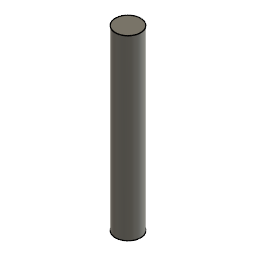
OTIS model assembly (Autodesk Fusion 360 archive; units mm, degrees)
design "Front wheel shaft"
part number: 2026-08-01-14-16-07-346
Autodesk Fusion 360 part; units mm, degrees
sketch "Sketch1" plane through (0, 0, 0) normal (0, 1, 0) x (1, 0, 0)
  circle A0 centre (0, 0) radius 1
  dimension "d1" = 2
  constraint coincident A0.centre origin
  measures "d1" diameter of A0
extrude "Extrude1" add sketch "Sketch1" along normal blind 14

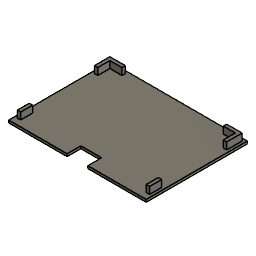
design "OTIS roof"
part number: 2026-08-06-09-41-14-601
Autodesk Fusion 360 part; units mm, degrees
sketch "Sketch1" plane through (0, 0, 0) normal (0, 1, 0) x (1, 0, 0)
  line L0 (0, 0) -> (80, 0)
  line L1 (80, 0) -> (80, 58.89)
  line L2 (80, 58.89) -> (0, 58.89)
  line L3 (0, 58.89) -> (0, 0)
  line L4 (46, 0) -> (34, 0)
  line L5 (34, 0) -> (34, 8)
  line L6 (34, 8) -> (46, 8)
  line L7 (46, 8) -> (46, 0)
  dimension "d1" = 58.89
  dimension "d2" = 80
  dimension "d11" = 8
  dimension "d14" = 12
  dimension "d15" = 34
  constraint horizontal L0
  constraint vertical L1
  constraint horizontal L2
  constraint vertical L3
  constraint coincident L0.start L3.end
  constraint horizontal L4
  constraint vertical L5
  constraint horizontal L6
  constraint vertical L7
  constraint coincident L0 L4.start
  measures "d1" distance of L0.start L2.end
  measures "d2" distance of L1 L3
  measures "d11" distance of L4.end L5.end
  measures "d14" distance of L5.end L6.end
  measures "d15" distance of L3 L5
extrude "Extrude1" add sketch "Sketch1" along normal blind 1.5
sketch "Sketch2" plane through (0, 1.5, 0) normal (0, 1, 0) x (-1, 0, 0)
  line L0 (0, -58.89) -> (0, 0)
  line L1 (0, 0) -> (-80, 0)
  line L2 (-80, 0) -> (-80, -58.89)
  line L3 (-80, -58.89) -> (0, -58.89)
  line L4 (-10.51, -1.51) -> (-1.51, -1.51)
  line L5 (-1.51, -1.51) -> (-1.51, -10.51)
  line L6 (-1.51, -10.51) -> (-10.51, -10.51)
  line L7 (-10.51, -10.51) -> (-10.51, -1.51)
  line L8 (-10.51, -10.51) -> (-3.51, -10.51)
  line L9 (-3.51, -10.51) -> (-3.51, -3.51)
  line L10 (-3.51, -3.51) -> (-10.51, -3.51)
  line L11 (-10.51, -3.51) -> (-10.51, -10.51)
  line L12 (0, -29.445) -> (-80, -29.445) construction
  line L13 (-3.51, -48.38) -> (-3.51, -55.38)
  line L14 (-3.51, -55.38) -> (-10.51, -55.38)
  line L15 (-10.51, -48.38) -> (-10.51, -57.38)
  line L16 (-1.51, -48.38) -> (-10.51, -48.38)
  line L17 (-1.51, -57.38) -> (-1.51, -48.38)
  line L18 (-10.51, -57.38) -> (-1.51, -57.38)
  line L19 (-69.49, -1.51) -> (-78.49, -1.51)
  line L20 (-76.49, -3.51) -> (-69.49, -3.51)
  line L21 (-78.49, -1.51) -> (-78.49, -10.51)
  line L22 (-76.49, -10.51) -> (-76.49, -3.51)
  line L23 (-78.49, -10.51) -> (-69.49, -10.51)
  line L24 (-69.49, -10.51) -> (-69.49, -1.51)
  line L25 (-78.49, -48.38) -> (-69.49, -48.38)
  line L26 (-69.49, -48.38) -> (-69.49, -57.38)
  line L27 (-76.49, -48.38) -> (-76.49, -55.38)
  line L28 (-78.49, -57.38) -> (-78.49, -48.38)
  line L29 (-76.49, -55.38) -> (-69.49, -55.38)
  line L30 (-69.49, -57.38) -> (-78.49, -57.38)
  line L31 (-3.51, -3.51) -> (-1.51, -3.51)
  line L32 (-76.49, -3.51) -> (-78.49, -3.51)
  dimension "d5" = 9
  dimension "d6" = 9
  dimension "d7" = 1.51
  dimension "d8" = 1.51
  constraint horizontal L4
  constraint vertical L5
  constraint horizontal L6
  constraint vertical L7
  constraint horizontal L8
  constraint vertical L9
  constraint horizontal L10
  constraint vertical L11
  constraint coincident L5 L31.end
  constraint perpendicular L9 L31
  constraint coincident L21 L32.end
  constraint perpendicular L21 L32
  measures "d5" distance of L4.start L4.end
  measures "d6" distance of L4.start L6.end
  measures "d7" distance of L0 L5
  measures "d8" distance of L1 L4
extrude "Extrude2" add sketch "Sketch2" along normal blind 4 contours L5 L6 L9 L31 | L13 L14 L15 L16 L17 L18 | L21 L22 L23 L32 | L25 L26 L27 L28 L29 L30
extrude "Extrude3" cut sketch "Sketch1" along normal blind 8.263 contours L0 L4 L5 L6 L7

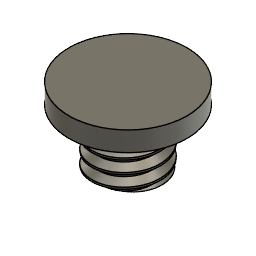
design "M2.5 x 6mm Phillips Flat Head Screw"
part number: 2026-08-01-20-11-09-453
Autodesk Fusion 360 part; units mm, degrees
sketch "Sketch1" plane through (0, 0, 0) normal (0, 1, 0) x (1, 0, 0)
  circle A0 centre (0, 0) radius 1.5
  dimension "d1" = 3
  constraint coincident A0.centre origin
  measures "d1" diameter of A0
extrude "Extrude1" add sketch "Sketch1" along normal blind 2
thread "Thread1" "ISO Metric profile 2.5 M2.5x0.45 M2.5x0.45 6g" major diameter 2.43 minor diameter 1.9165 pitch 0.45 angle 60 modelled right hand crest width 0.0648 on face at (1.4981, 1.3333, 0.0748) crest through (1.215, -0.1125, 0)
sketch "Sketch2" plane through (0, 2, 0) normal (0, 1, 0) x (-1, 0, 0)
  spline S0 degree 3 poles (-0.1252, 1.2085) (-0.2764, 1.1771) (-0.4201, 1.117) (-0.6707, 0.9476) (-0.7764, 0.8419) (-0.9369, 0.6004) (-0.9921, 0.4683) (-1.0464, 0.1962) (-1.0473, 0.0593) (-1.0042, -0.1619) (-0.9753, -0.2474) (-0.8966, -0.4057) (-0.8477, -0.4781) (-0.7897, -0.5428) knots 0 0 0 0 0.046326 0.046326 0.090815 0.090815 0.133466 0.133466 0.17428 0.17428 0.201332 0.201332 0.227524 0.227524 0.227524 0.227524
  arc A0 (-0.7897, -0.5428) -> (0.2561, -0.9234) centre (0, 0) ccw
  spline S1 degree 3 poles (0.2561, -0.9234) (0.3815, -0.9055) (0.5022, -0.8627) (0.7262, -0.7312) (0.8263, -0.6416) (0.9913, -0.4249) (1.0527, -0.2985) (1.1264, -0.0233) (1.1356, 0.1233) (1.1038, 0.3714) (1.0763, 0.4727) (0.9942, 0.6681) (0.9393, 0.7609) (0.8727, 0.8453) knots 0 0 0 0 0.038021 0.038021 0.077873 0.077873 0.119555 0.119555 0.163068 0.163068 0.19429 0.19429 0.22638 0.22638 0.22638 0.22638
  arc A1 (0.8727, 0.8453) -> (-0.1252, 1.2085) centre (0, 0) ccw
  circle A2 centre (0, 0) radius 2.1
  dimension "d6" = 4.2
  constraint coincident A0.centre A1.centre
  measures "d6" diameter of A2
extrude "Extrude2" add sketch "Sketch2" along normal blind 0.7 contours S0 A0 S1 A1 | A2

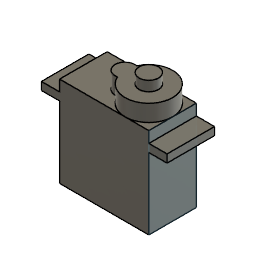
design "MG90S servo model"
part number: 2026-07-24-13-32-31-393
Autodesk Fusion 360 part; units mm, degrees
sketch "Sketch1" plane through (0, 0, 0) normal (0, 1, 0) x (1, 0, 0)
  line L0 (0, 0) -> (22.5, 0)
  line L1 (22.5, 0) -> (22.5, 12)
  line L2 (22.5, 12) -> (0, 12)
  line L3 (0, 12) -> (0, 0)
  dimension "d1" = 22.5
  dimension "d2" = 12
  constraint horizontal L0
  constraint vertical L1
  constraint horizontal L2
  constraint vertical L3
  constraint coincident L0.start L3.end
  measures "d1" distance of L0.start L0.end
  measures "d2" distance of L0.start L2.end
extrude "Extrude1" add sketch "Sketch1" along normal blind 22.8
sketch "Sketch2" plane through (22.5, 0, 0) normal (1, 0, 0) x (0, 0, -1)
  line L0 (0, 0) -> (12, 0)
  line L1 (12, 0) -> (12, 22.8)
  line L2 (12, 22.8) -> (0, 22.8)
  line L3 (0, 22.8) -> (0, 0)
sketch "Sketch3" plane through (0, 22.8, 0) normal (0, 1, 0) x (-1, 0, 0)
  line L0 (0, -12) -> (0, 0)
  line L1 (0, 0) -> (-22.5, 0)
  line L2 (-22.5, 0) -> (-22.5, -12)
  line L3 (-22.5, -12) -> (0, -12)
  line L4 (-22.5, -6) -> (-16.5, -6) construction
  circle A0 centre (-16.5, -6) radius 6
  line L5 (-16.5, -6) -> (0, -6) construction
  circle A1 centre (-10.5, -6) radius 2.5
  dimension "d5" = 6
  dimension "d6" = 12
  dimension "d16" = 5
  constraint midpoint L2 L4.start
  constraint perpendicular L2 L4
  constraint coincident L4.end A0.centre
  constraint midpoint L0 L5.end
  constraint coincident A0 A1.centre
  constraint coincident L5 A1.centre
  measures "d5" distance of L4.start L4.end
  measures "d6" diameter of A0
  measures "d16" diameter of A1
extrude "Extrude2" add sketch "Sketch3" along normal blind 4.2 contours A0 A1 | A0 A1 | A0 A1
sketch "Sketch4" plane through (0, 27, 0) normal (0, 1, 0) x (-1, 0, 0)
  arc A0 (-11.0208, -8.4451) -> (-11.0208, -3.5549) centre (-10.5, -6) ccw
  arc A1 (-11.0208, -3.5549) -> (-11.0208, -8.4451) centre (-16.5, -6) ccw
  circle A2 centre (-16.5, -6) radius 2.45
  dimension "d17" = 4.9
  constraint concentric A1 A2
  measures "d17" diameter of A2
sketch "Sketch5" plane through (22.5, 0, 0) normal (1, 0, 0) x (0, 0, -1)
  line L0 (12, 18) -> (0, 18)
  line L1 (0, 18) -> (0, 20)
  line L2 (0, 20) -> (12, 20)
  line L3 (12, 20) -> (12, 18)
  constraint horizontal L0
  constraint vertical L1
  constraint horizontal L2
  constraint vertical L3
extrude "Extrude4" add sketch "Sketch5" along normal blind 4.6
sketch "Sketch8" plane through (0, 0, 0) normal (-1, 0, 0) x (0, 0, 1)
  line L0 (-12, 0) -> (0, 0)
  line L1 (0, 0) -> (0, 22.8)
  line L2 (0, 22.8) -> (-12, 22.8)
  line L3 (-12, 22.8) -> (-12, 0)
  line L4 (-12, 20) -> (0, 20)
  line L5 (0, 20) -> (0, 18)
  line L6 (0, 18) -> (-12, 18)
  line L7 (-12, 18) -> (-12, 20)
extrude "Extrude5" add sketch "Sketch8" along normal blind 4.6 contours L1 L3 L4 L5 L6 L7
extrude "Extrude6" add sketch "Sketch4" along normal blind 2.5 contours A2

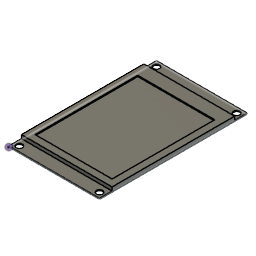
design "rough 2.4 in lcd model"
part number: 2026-07-24-14-02-43-553
Autodesk Fusion 360 part; units mm, degrees
sketch "Sketch1" plane through (0, 0, 0) normal (0, 1, 0) x (1, 0, 0)
  line L0 (0, 0) -> (43.3, 0)
  line L1 (43.3, 0) -> (43.3, 70.5)
  line L2 (43.3, 70.5) -> (0, 70.5)
  line L3 (0, 70.5) -> (0, 0)
  dimension "d1" = 43.3
  dimension "d2" = 70.5
  constraint horizontal L0
  constraint vertical L1
  constraint horizontal L2
  constraint vertical L3
  constraint coincident L0.start L3.end
  measures "d1" distance of L0.start L0.end
  measures "d2" distance of L0.start L2.end
extrude "Extrude1" add sketch "Sketch1" along normal blind 0.5
sketch "Sketch2" plane through (0, 0.5, 0) normal (0, 1, 0) x (-1, 0, 0)
  line L0 (0, -70.5) -> (0, 0)
  line L1 (0, 0) -> (-43.3, 0)
  line L2 (-43.3, 0) -> (-43.3, -70.5)
  line L3 (-43.3, -70.5) -> (0, -70.5) construction
  line L4 (-43.3, 0) -> (-43.3, -5) construction
  line L5 (-43.3, -70.5) -> (-43.3, -64.5) construction
  line L6 (-43.3, -64.5) -> (0, -64.5)
  line L7 (0, -64.5) -> (0, -6)
  line L8 (0, -6) -> (-43.3, -6)
  line L9 (-43.3, -6) -> (-43.3, -64.5)
  line L10 (0, -2.5) -> (-2.5, -2.5) construction
  line L11 (-43.3, -2.5) -> (-40.8, -2.5) construction
  circle A0 centre (-2.5, -68) radius 1.5
  circle A1 centre (-40.8, -68) radius 1.5
  circle A2 centre (-40.8, -2.5) radius 1.5
  circle A3 centre (-2.5, -2.5) radius 1.5
  dimension "d5" = 6
  dimension "d8" = 2.5
  dimension "d10" = 3
  dimension "d11" = 3
  dimension "d12" = 3
  dimension "d13" = 3
  dimension "d16" = 2.5
  dimension "d17" = 2.5
  dimension "d18" = 2.5
  dimension "d19" = 2.5
  dimension "d20" = 2.5
  dimension "d21" = 2.5
  dimension "d22" = 2.5
  constraint coincident L1.end L2.start
  constraint coincident L2 L4.end
  constraint coincident L2.end L3.start
  constraint perpendicular L3 L5
  constraint horizontal L6
  constraint vertical L7
  constraint horizontal L8
  constraint vertical L9
  constraint coincident L0 L7.end
  constraint coincident L0 L10.start
  constraint perpendicular L0 L10
  constraint midpoint L4 L11.start
  constraint perpendicular L4 L11
  constraint coincident L11.end A2.centre
  constraint coincident L10.end A3.centre
  measures "d5" distance of L2.end L5.end
  measures "d8" distance of L11.start L11.end
  measures "d10" diameter of A0
  measures "d11" diameter of A1
  measures "d12" diameter of A2
  measures "d13" diameter of A3
  measures "d16" distance of L10.start L10.end
  measures "d17" distance of L1 L10.end
  measures "d18" distance of L1 L11.end
  measures "d19" distance of L5 A1.centre
  measures "d20" distance of L3 A1.centre
  measures "d21" distance of L3 A0.centre
  measures "d22" distance of L0 A0.centre
extrude "Extrude2" add sketch "Sketch2" along normal blind 1.67 contours L0 L2 L6 L7 L8 L9
extrude "Extrude3" cut sketch "Sketch2" against normal blind 5.737 contours A0 | A1 | A2 | A3
sketch "Sketch3" plane through (0, 2.17, 0) normal (0, 1, 0) x (-1, 0, 0)
  line L0 (-43.3, -6) -> (-43.3, -64.5)
  line L1 (-43.3, -64.5) -> (0, -64.5)
  line L2 (0, -64.5) -> (0, -6)
  line L3 (0, -6) -> (-43.3, -6)
  line L4 (-3.29, -9.29) -> (-40.01, -9.29)
  line L5 (-40.01, -9.29) -> (-40.01, -58.25)
  line L6 (-40.01, -58.25) -> (-3.29, -58.25)
  line L7 (-3.29, -58.25) -> (-3.29, -9.29)
  dimension "d23" = 36.72
  dimension "d24" = 48.96
  dimension "d25" = 3.29
  dimension "d26" = 3.29
  constraint horizontal L4
  constraint vertical L5
  constraint horizontal L6
  constraint vertical L7
  measures "d23" distance of L4.start L4.end
  measures "d24" distance of L4.start L6.end
  measures "d25" distance of L3 L4
  measures "d26" distance of L0 L5
extrude "Extrude4" cut sketch "Sketch3" against normal blind 0.5 contours L4 L5 L6 L7

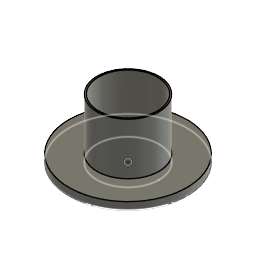
design "Front wheel shaft stopper"
part number: 2026-08-01-14-29-53-919
Autodesk Fusion 360 part; units mm, degrees
sketch "Sketch1" plane through (0, 0, 0) normal (0, 1, 0) x (1, 0, 0)
  circle A0 centre (0, 0) radius 2
  circle A1 centre (0, 0) radius 1.05
  dimension "d1" = 4
  dimension "d2" = 2.1
  constraint coincident A0.centre A1.centre
  measures "d1" diameter of A0
  measures "d2" diameter of A1
extrude "Extrude1" add sketch "Sketch1" along normal blind 0.25
extrude "Extrude2" add sketch "Sketch1" along normal blind 2 contours A1
sketch "Sketch2" plane through (0, 0, 0) normal (0, 1, 0) x (1, 0, 0)
  circle A0 centre (0, 0) radius 1
  dimension "d8" = 2
  constraint coincident A0.centre origin
  measures "d8" diameter of A0
extrude "Extrude3" cut sketch "Sketch2" along normal blind 3.883

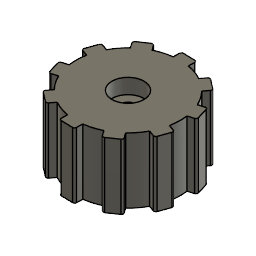
design "Tank tread gear"
part number: 2026-08-01-11-00-48-314
Autodesk Fusion 360 part; units mm, degrees
sketch "Sketch1" plane through (0, 0, 0) normal (0, 1, 0) x (1, 0, 0)
  circle A0 centre (0, 0) radius 8
  line L0 (1.3935, 7.8777) -> (1.4168, 8.8274)
  line L1 (1.1242, 9.1347) -> (-0.6752, 9.1788)
  line L2 (-0.9825, 8.8862) -> (-1.0058, 7.9365)
  line L3 (-3.503, 7.1923) -> (-4.0424, 7.9743)
  line L4 (-4.4597, 8.0509) -> (-5.9414, 7.0289)
  line L5 (-6.018, 6.6116) -> (-5.4786, 5.8296)
  line L6 (-7.0615, 3.7597) -> (-7.9575, 4.0753)
  line L7 (-8.3402, 3.892) -> (-8.9382, 2.1942)
  line L8 (-8.7549, 1.8116) -> (-7.8589, 1.496)
  line L9 (-7.9228, -1.109) -> (-8.8332, -1.3804)
  line L10 (-9.035, -1.7535) -> (-8.5209, -3.4786)
  line L11 (-8.1477, -3.6804) -> (-7.2373, -3.4091)
  line L12 (-5.7578, -5.5541) -> (-6.3348, -6.3087)
  line L13 (-6.2788, -6.7293) -> (-4.8489, -7.8227)
  line L14 (-4.4284, -7.7666) -> (-3.8513, -7.012)
  line L15 (-1.3935, -7.8777) -> (-1.4168, -8.8274)
  line L16 (-1.1242, -9.1347) -> (0.6752, -9.1788)
  line L17 (0.9825, -8.8862) -> (1.0058, -7.9365)
  line L18 (3.503, -7.1923) -> (4.0424, -7.9743)
  line L19 (4.4597, -8.0509) -> (5.9414, -7.0289)
  line L20 (6.018, -6.6116) -> (5.4786, -5.8296)
  line L21 (7.0615, -3.7597) -> (7.9575, -4.0753)
  line L22 (8.3402, -3.892) -> (8.9382, -2.1942)
  line L23 (8.7549, -1.8116) -> (7.8589, -1.496)
  line L24 (7.9228, 1.109) -> (8.8332, 1.3804)
  line L25 (9.035, 1.7535) -> (8.5209, 3.4786)
  line L26 (8.1477, 3.6804) -> (7.2373, 3.4091)
  line L27 (5.7578, 5.5541) -> (6.3348, 6.3087)
  line L28 (6.2788, 6.7293) -> (4.8489, 7.8227)
  line L29 (4.4284, 7.7666) -> (3.8513, 7.012)
  arc A1 (-0.6752, 9.1788) -> (-0.9825, 8.8862) centre (-0.6826, 8.8789) ccw
  arc A2 (1.4168, 8.8274) -> (1.1242, 9.1347) centre (1.1169, 8.8348) ccw
  arc A3 (4.8489, 7.8227) -> (4.4284, 7.7666) centre (4.6667, 7.5844) ccw
  arc A4 (6.3348, 6.3087) -> (6.2788, 6.7293) centre (6.0965, 6.491) ccw
  arc A5 (8.5209, 3.4786) -> (8.1477, 3.6804) centre (8.2334, 3.3929) ccw
  arc A6 (8.8332, 1.3804) -> (9.035, 1.7535) centre (8.7475, 1.6679) ccw
  arc A7 (8.9382, -2.1942) -> (8.7549, -1.8116) centre (8.6552, -2.0946) ccw
  arc A8 (7.9575, -4.0753) -> (8.3402, -3.892) centre (8.0572, -3.7923) ccw
  arc A9 (5.9414, -7.0289) -> (6.018, -6.6116) centre (5.7711, -6.782) ccw
  arc A10 (4.0424, -7.9743) -> (4.4597, -8.0509) centre (4.2894, -7.804) ccw
  arc A11 (0.6752, -9.1788) -> (0.9825, -8.8862) centre (0.6826, -8.8789) ccw
  arc A12 (-1.4168, -8.8274) -> (-1.1242, -9.1347) centre (-1.1169, -8.8348) ccw
  arc A13 (-4.8489, -7.8227) -> (-4.4284, -7.7666) centre (-4.6667, -7.5844) ccw
  arc A14 (-6.3348, -6.3087) -> (-6.2788, -6.7293) centre (-6.0965, -6.491) ccw
  arc A15 (-8.5209, -3.4786) -> (-8.1477, -3.6804) centre (-8.2334, -3.3929) ccw
  arc A16 (-8.8332, -1.3804) -> (-9.035, -1.7535) centre (-8.7475, -1.6679) ccw
  arc A17 (-7.9575, 4.0753) -> (-8.3402, 3.892) centre (-8.0572, 3.7923) ccw
  arc A18 (-8.9382, 2.1942) -> (-8.7549, 1.8116) centre (-8.6552, 2.0946) ccw
  arc A19 (-4.0424, 7.9743) -> (-4.4597, 8.0509) centre (-4.2894, 7.804) ccw
  arc A20 (-5.9414, 7.0289) -> (-6.018, 6.6116) centre (-5.7711, 6.782) ccw
  point P0 (-0.9751, 9.1862)
  dimension "d1" = 16
  dimension "d2" = 2.4
  dimension "d3" = 1.25
  dimension "d6" = 0.3
  constraint coincident A0.centre origin
  constraint coincident A0 L2.end
  constraint coincident A0 L0.start
  constraint parallel L0 L2
  constraint perpendicular L1 L2
  constraint coincident P0 L1
  constraint coincident P0 L2
  constraint tangent L1 A1
  constraint tangent L2 A1
  constraint tangent L0 A2
  constraint tangent L1 A2
  constraint equal A1 A2
  constraint tangent L28 A3
  constraint tangent L29 A3
  constraint equal A1 A3
  constraint tangent L27 A4
  constraint tangent L28 A4
  constraint equal A1 A4
  constraint tangent L25 A5
  constraint tangent L26 A5
  constraint equal A1 A5
  constraint tangent L24 A6
  constraint tangent L25 A6
  constraint equal A1 A6
  constraint tangent L22 A7
  constraint tangent L23 A7
  constraint equal A1 A7
  constraint tangent L21 A8
  constraint tangent L22 A8
  constraint equal A1 A8
  constraint tangent L19 A9
  constraint tangent L20 A9
  constraint equal A1 A9
  constraint tangent L18 A10
  constraint tangent L19 A10
  constraint equal A1 A10
  constraint tangent L16 A11
  constraint tangent L17 A11
  constraint equal A1 A11
  constraint tangent L15 A12
  constraint tangent L16 A12
  constraint equal A1 A12
  constraint tangent L13 A13
  constraint tangent L14 A13
  constraint equal A1 A13
  constraint tangent L12 A14
  constraint tangent L13 A14
  constraint equal A1 A14
  constraint tangent L10 A15
  constraint tangent L11 A15
  constraint equal A1 A15
  constraint tangent L9 A16
  constraint tangent L10 A16
  constraint equal A1 A16
  constraint tangent L6 A17
  constraint tangent L7 A17
  constraint equal A1 A17
  constraint tangent L7 A18
  constraint tangent L8 A18
  constraint equal A1 A18
  constraint tangent L3 A19
  constraint tangent L4 A19
  constraint equal A1 A19
  constraint tangent L4 A20
  constraint tangent L5 A20
  constraint equal A1 A20
  measures "d1" diameter of A0
  measures "d2" distance of L2.end L0.start
  measures "d3" distance of L2.end P0
  measures "d6" radius of A1
extrude "Extrude1" add sketch "Sketch1" along normal blind 10
sketch "Sketch2" plane through (0, 10, 0) normal (0, 1, 0) x (-1, 0, 0)
  arc A0 (5.9414, -7.0289) -> (6.018, -6.6116) centre (5.7711, -6.782) ccw
  line L0 (6.018, -6.6116) -> (5.4786, -5.8296)
  arc A1 (5.4786, -5.8296) -> (7.0615, -3.7597) centre (0, 0) ccw
  line L1 (7.0615, -3.7597) -> (7.9575, -4.0753)
  arc A2 (7.9575, -4.0753) -> (8.3402, -3.892) centre (8.0572, -3.7923) ccw
  line L2 (8.3402, -3.892) -> (8.9382, -2.1942)
  arc A3 (8.9382, -2.1942) -> (8.7549, -1.8116) centre (8.6552, -2.0946) ccw
  line L3 (8.7549, -1.8116) -> (7.8589, -1.496)
  arc A4 (7.8589, -1.496) -> (7.9228, 1.109) centre (0, 0) ccw
  line L4 (7.9228, 1.109) -> (8.8332, 1.3804)
  arc A5 (8.8332, 1.3804) -> (9.035, 1.7535) centre (8.7475, 1.6679) ccw
  line L5 (9.035, 1.7535) -> (8.5209, 3.4786)
  arc A6 (8.5209, 3.4786) -> (8.1477, 3.6804) centre (8.2334, 3.3929) ccw
  line L6 (8.1477, 3.6804) -> (7.2373, 3.4091)
  arc A7 (7.2373, 3.4091) -> (5.7578, 5.5541) centre (0, 0) ccw
  line L7 (5.7578, 5.5541) -> (6.3348, 6.3087)
  arc A8 (6.3348, 6.3087) -> (6.2788, 6.7293) centre (6.0965, 6.491) ccw
  line L8 (6.2788, 6.7293) -> (4.8489, 7.8227)
  arc A9 (4.8489, 7.8227) -> (4.4284, 7.7666) centre (4.6667, 7.5844) ccw
  line L9 (4.4284, 7.7666) -> (3.8513, 7.012)
  arc A10 (3.8513, 7.012) -> (1.3935, 7.8777) centre (0, 0) ccw
  line L10 (1.3935, 7.8777) -> (1.4168, 8.8274)
  arc A11 (1.4168, 8.8274) -> (1.1242, 9.1347) centre (1.1169, 8.8348) ccw
  line L11 (1.1242, 9.1347) -> (-0.6752, 9.1788)
  arc A12 (-0.6752, 9.1788) -> (-0.9825, 8.8862) centre (-0.6826, 8.8789) ccw
  line L12 (-0.9825, 8.8862) -> (-1.0058, 7.9365)
  arc A13 (-1.0058, 7.9365) -> (-3.503, 7.1923) centre (0, 0) ccw
  line L13 (-3.503, 7.1923) -> (-4.0424, 7.9743)
  arc A14 (-4.0424, 7.9743) -> (-4.4597, 8.0509) centre (-4.2894, 7.804) ccw
  line L14 (-4.4597, 8.0509) -> (-5.9414, 7.0289)
  arc A15 (-5.9414, 7.0289) -> (-6.018, 6.6116) centre (-5.7711, 6.782) ccw
  line L15 (-6.018, 6.6116) -> (-5.4786, 5.8296)
  arc A16 (-5.4786, 5.8296) -> (-7.0615, 3.7597) centre (0, 0) ccw
  line L16 (-7.0615, 3.7597) -> (-7.9575, 4.0753)
  arc A17 (-7.9575, 4.0753) -> (-8.3402, 3.892) centre (-8.0572, 3.7923) ccw
  line L17 (-8.3402, 3.892) -> (-8.9382, 2.1942)
  arc A18 (-8.9382, 2.1942) -> (-8.7549, 1.8116) centre (-8.6552, 2.0946) ccw
  line L18 (-8.7549, 1.8116) -> (-7.8589, 1.496)
  arc A19 (-7.8589, 1.496) -> (-7.9228, -1.109) centre (0, 0) ccw
  line L19 (-7.9228, -1.109) -> (-8.8332, -1.3804)
  arc A20 (-8.8332, -1.3804) -> (-9.035, -1.7535) centre (-8.7475, -1.6679) ccw
  line L20 (-9.035, -1.7535) -> (-8.5209, -3.4786)
  arc A21 (-8.5209, -3.4786) -> (-8.1477, -3.6804) centre (-8.2334, -3.3929) ccw
  line L21 (-8.1477, -3.6804) -> (-7.2373, -3.4091)
  arc A22 (-7.2373, -3.4091) -> (-5.7578, -5.5541) centre (0, 0) ccw
  line L22 (-5.7578, -5.5541) -> (-6.3348, -6.3087)
  arc A23 (-6.3348, -6.3087) -> (-6.2788, -6.7293) centre (-6.0965, -6.491) ccw
  line L23 (-6.2788, -6.7293) -> (-4.8489, -7.8227)
  arc A24 (-4.8489, -7.8227) -> (-4.4284, -7.7666) centre (-4.6667, -7.5844) ccw
  line L24 (-4.4284, -7.7666) -> (-3.8513, -7.012)
  arc A25 (-3.8513, -7.012) -> (-1.3935, -7.8777) centre (0, 0) ccw
  line L25 (-1.3935, -7.8777) -> (-1.4168, -8.8274)
  arc A26 (-1.4168, -8.8274) -> (-1.1242, -9.1347) centre (-1.1169, -8.8348) ccw
  line L26 (-1.1242, -9.1347) -> (0.6752, -9.1788)
  arc A27 (0.6752, -9.1788) -> (0.9825, -8.8862) centre (0.6826, -8.8789) ccw
  line L27 (0.9825, -8.8862) -> (1.0058, -7.9365)
  arc A28 (1.0058, -7.9365) -> (3.503, -7.1923) centre (0, 0) ccw
  line L28 (3.503, -7.1923) -> (4.0424, -7.9743)
  arc A29 (4.0424, -7.9743) -> (4.4597, -8.0509) centre (4.2894, -7.804) ccw
  line L29 (4.4597, -8.0509) -> (5.9414, -7.0289)
  circle A30 centre (0, 0) radius 2.45
  dimension "d9" = 4.9
  constraint concentric A1 A30
  measures "d9" diameter of A30
extrude "Extrude2" cut sketch "Sketch2" against normal blind 2.3 contours A30
sketch "Sketch3" plane through (0, 7.7, 0) normal (0, 1, 0) x (-1, 0, 0)
  circle A0 centre (0, 0) radius 2.45
  circle A1 centre (0, 0) radius 1.05
  dimension "d12" = 2.1
  constraint concentric A0 A1
  measures "d12" diameter of A1
extrude "Extrude3" cut sketch "Sketch3" against normal blind 44.519 contours A1

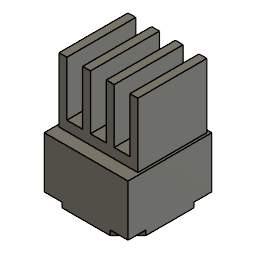
design "Camera Module"
part number: 2026-08-01-18-53-29-409
Autodesk Fusion 360 part; units mm, degrees
sketch "Sketch1" plane through (0, 0, 0) normal (0, 1, 0) x (1, 0, 0)
  line L0 (0, 0) -> (8.5, 0)
  line L1 (8.5, 0) -> (8.5, 8.5)
  line L2 (8.5, 8.5) -> (0, 8.5)
  line L3 (0, 8.5) -> (0, 0)
  dimension "d1" = 8.5
  dimension "d2" = 8.5
  constraint horizontal L0
  constraint vertical L1
  constraint horizontal L2
  constraint vertical L3
  constraint coincident L0.start L3.end
  measures "d1" distance of L0.start L0.end
  measures "d2" distance of L0.start L2.end
extrude "Extrude1" add sketch "Sketch1" along normal blind 5.2
sketch "Sketch2" plane through (0, 5.2, 0) normal (0, 1, 0) x (-1, 0, 0)
  line L0 (0, -8.5) -> (0, 0)
  line L1 (0, 0) -> (-8.5, 0)
  line L2 (-8.5, 0) -> (-8.5, -8.5)
  line L3 (-8.5, -8.5) -> (0, -8.5)
  line L4 (-0.25, -8.25) -> (-8.25, -8.25)
  line L5 (-8.25, -8.25) -> (-8.25, -1.25)
  line L6 (-8.25, -1.25) -> (-0.25, -1.25)
  line L7 (-0.25, -1.25) -> (-0.25, -8.25)
  dimension "d5" = 8
  dimension "d6" = 7
  dimension "d7" = 0.25
  dimension "d8" = 0.25
  constraint horizontal L4
  constraint vertical L5
  constraint horizontal L6
  constraint vertical L7
  measures "d5" distance of L4.start L4.end
  measures "d6" distance of L4.start L6.end
  measures "d7" distance of L2 L5
  measures "d8" distance of L3 L4
sketch "Sketch3" plane through (0, 5.2, 0) normal (0, 1, 0) x (-1, 0, 0)
extrude "Extrude2" add sketch "Sketch2" along normal blind 1 contours L4 L5 L6 L7
sketch "Sketch4" plane through (0, 6.2, 0) normal (0, 1, 0) x (-1, 0, 0)
  line L0 (-0.25, -1.25) -> (-8.25, -1.25)
  line L1 (-8.25, -1.25) -> (-8.25, -8.25)
  line L2 (-8.25, -8.25) -> (-0.25, -8.25)
  line L3 (-0.25, -8.25) -> (-0.25, -1.25)
  line L4 (-0.25, -8.25) -> (-1.05, -8.25)
  line L5 (-1.05, -8.25) -> (-1.05, -1.25)
  line L6 (-1.05, -1.25) -> (-0.25, -1.25)
  line L7 (-0.25, -1.25) -> (-0.25, -8.25)
  line L8 (-2.65, -8.25) -> (-3.45, -8.25)
  line L9 (-2.65, -1.25) -> (-2.65, -8.25)
  line L10 (-3.45, -8.25) -> (-3.45, -1.25)
  line L11 (-3.45, -1.25) -> (-2.65, -1.25)
  line L12 (-5.05, -8.25) -> (-5.85, -8.25)
  line L13 (-5.05, -1.25) -> (-5.05, -8.25)
  line L14 (-5.85, -8.25) -> (-5.85, -1.25)
  line L15 (-5.85, -1.25) -> (-5.05, -1.25)
  line L16 (-7.45, -8.25) -> (-8.25, -8.25)
  line L17 (-7.45, -1.25) -> (-7.45, -8.25)
  line L18 (-8.25, -8.25) -> (-8.25, -1.25)
  line L19 (-8.25, -1.25) -> (-7.45, -1.25)
  dimension "d11" = 0.8
  dimension "d12" = 7
  dimension "d15" = -7.2
  dimension "d16" = 0
  constraint horizontal L4
  constraint vertical L5
  constraint horizontal L6
  constraint vertical L7
  constraint coincident L2.end L3.start
  measures "d11" distance of L2.end L4.end
  measures "d12" distance of L2.end L0.start
extrude "Extrude3" add sketch "Sketch4" along normal blind 5.519 contours L0 L2 L3 L4 L5 L6 L7 | L0 L2 L8 L9 L10 L11 | L0 L2 L12 L13 L14 L15 | L0 L1 L2 L16 L17 L18 L19
sketch "Sketch5" plane through (0, 0, 0) normal (0, -1, 0) x (1, 0, 0)
  line L0 (0, 0) -> (0, -8.5)
  line L1 (0, -8.5) -> (8.5, -8.5)
  line L2 (8.5, -8.5) -> (8.5, 0)
  line L3 (8.5, 0) -> (0, 0)
  line L4 (6.7, -8.5) -> (1.8, -8.5)
  line L5 (0, -6.7) -> (0, -1.8)
  line L6 (1.8, 0) -> (6.7, 0)
  line L7 (8.5, -1.8) -> (8.5, -6.7)
  line L8 (0, -1.8) -> (1.8, 0)
  line L9 (6.7, 0) -> (8.5, -1.8)
  line L10 (1.8, -8.5) -> (0, -6.7)
  line L11 (6.7, -8.5) -> (8.5, -6.7)
  point P0 (8.5, -8.5)
  point P1 (0, -8.5)
  point P2 (8.5, 0)
  dimension "d19" = 8.5
  dimension "d20" = 8.5
  dimension "d23" = 1.8
  dimension "d24" = 1.8
  dimension "d25" = 1.8
  dimension "d26" = 1.8
  dimension "d27" = 1.8
  dimension "d28" = 1.8
  dimension "d29" = 1.8
  dimension "d30" = 1.8
  constraint horizontal L4
  constraint vertical L5
  constraint horizontal L6
  constraint vertical L7
  constraint coincident L0.start L5
  constraint coincident L0.start L6
  constraint coincident L2 L7
  constraint coincident P2 L6
  constraint coincident P2 L7
  constraint coincident P1 L4
  constraint coincident P1 L5
  constraint coincident P0 L4
  constraint coincident P0 L7
  measures "d19" distance of P0 P1
  measures "d20" distance of P1 L0.start
  measures "d23" distance of L0.start L5.end
  measures "d24" distance of L0.start L6.start
  measures "d25" distance of P2 L6.end
  measures "d26" distance of P2 L7.start
  measures "d27" distance of P1 L4.end
  measures "d28" distance of P1 L5.start
  measures "d29" distance of P0 L4.start
  measures "d30" distance of P0 L7.end
extrude "Extrude4" add sketch "Sketch5" along normal blind 0.5 contours L0 L1 L2 L3 L4 L5 L6 L7 L8 L9 L10 L11
sketch "Sketch6" plane through (0, -0.5, 0) normal (0, -1, 0) x (1, 0, 0)
  line L0 (1.8, -8.5) -> (6.7, -8.5)
  line L1 (6.7, -8.5) -> (8.5, -6.7)
  line L2 (8.5, -6.7) -> (8.5, -1.8)
  line L3 (8.5, -1.8) -> (6.7, 0)
  line L4 (6.7, 0) -> (1.8, 0)
  line L5 (1.8, 0) -> (0, -1.8)
  line L6 (0, -1.8) -> (0, -6.7)
  line L7 (0, -6.7) -> (1.8, -8.5)
  circle A0 centre (4.25, -4.25) radius 3.35
  dimension "d32" = 6.7
  measures "d32" diameter of A0
extrude "Extrude5" cut sketch "Sketch6" against normal blind 0.346 contours A0
equation "d24 = d23"

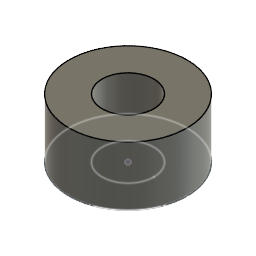
design "Front wheel shaft guide"
part number: 2026-08-01-14-11-48-809
Autodesk Fusion 360 part; units mm, degrees
sketch "Sketch1" plane through (0, 0, 0) normal (0, 1, 0) x (1, 0, 0)
  circle A0 centre (0, 0) radius 2.4
  circle A1 centre (0, 0) radius 1.05
  dimension "d1" = 4.8
  dimension "d2" = 2.1
  constraint coincident A0.centre A1.centre
  constraint concentric A0 A1
  measures "d1" diameter of A0
  measures "d2" diameter of A1
extrude "Extrude1" add sketch "Sketch1" along normal blind 2.4
